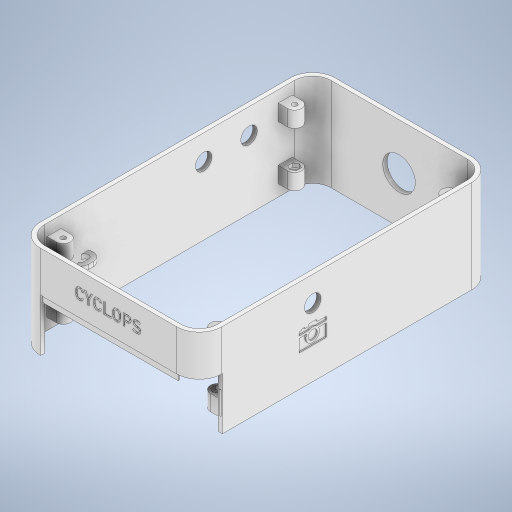
# Autodesk Inventor part: MIDDLE
Saved by Autodesk Inventor 2023 (Build 270158000, 158)
## iProperties
Created: 2023-03-14
Part Number: MIDDLE
Material: PC/ABS Plastic
Document SubType Name: Modeling
Designer: Amos Yu
Density: 0.357273 g/cm^3
Appearance: White
Author: Amos Yu
Autodesk Inventor part; units mm, degrees
note: some values were not read from the file. Chosen so that the rebuilt part matches the saved one: direction of "Hole2"; direction of "Hole3"; direction of "Hole4".
ref_plane "YZ Plane" through (0, 0, 0) normal (1, 0, 0) x (0, 1, 0)
sketch "Sketch1" plane through (0, 0, 0) normal (0, 1, 0) x (-1, 0, 0)
  line L0 (10, 0) -> (70, 0)
  line L1 (80, -10) -> (80, -120)
  line L2 (70, -130) -> (10, -130)
  line L3 (0, -120) -> (0, -10)
  arc A0 (80, -10) -> (70, 0) centre (70, -10) ccw
  arc A1 (10, 0) -> (0, -10) centre (10, -10) ccw
  arc A2 (0, -120) -> (10, -130) centre (10, -120) ccw
  arc A3 (70, -130) -> (80, -120) centre (70, -120) ccw
  line L4 (78.1, -120) -> (78.1, -10)
  arc A4 (78.1, -10) -> (70, -1.9) centre (70, -10) ccw
  line L5 (70, -1.9) -> (10, -1.9)
  arc A5 (10, -1.9) -> (1.9, -10) centre (10, -10) ccw
  line L6 (1.9, -10) -> (1.9, -120)
  arc A6 (1.9, -120) -> (10, -128.1) centre (10, -120) ccw
  line L7 (10, -128.1) -> (70, -128.1)
  arc A7 (70, -128.1) -> (78.1, -120) centre (70, -120) ccw
  point P0 (0, 0)
  point P1 (80, -130)
  point P2 (80, 0)
  point P3 (0, -130)
  dimension "d0" = 80
  dimension "d1" = 130
  dimension "d2" = 10
  dimension "d3" = 1.9
  constraints: 16 end point, 16 point on circle, 8 centre point, 8 point on line, 8 tangent, 4 parallel, 3 equal radius, 2 perpendicular, 1 horizontal, 7 other
  measures "d0" distance of point (80, -130) point (0, -130)
  measures "d1" distance of point (80, 0) point (80, -130)
  measures "d2" radius of A0
  measures "d3" distance between parallel lines of L1 L4
extrude "Extrusion1" add sketch "Sketch1" along normal mid plane 41
ref_plane "Work Plane1" through (0, -15.4, 0) normal (0, -1, 0) x (1, 0, 0)
sketch "Sketch2" plane through (0, -15.4, 0) normal (0, -1, 0) x (1, 0, 0)
  circle A0 centre (-6, -14) radius 1.1
  arc A1 (-6, -10.9) -> (-6, -17.1) centre (-6, -14) ccw
  line L0 (-6, -10.9) -> (-1.9, -10.9)
  line L1 (-1.9, -10.9) -> (-1.9, -17.1)
  line L2 (-1.9, -17.1) -> (-6, -17.1)
  line L3 (-1.9, -120) -> (-1.9, -10) projected
  circle A2 centre (-6, -116) radius 1.1
  arc A3 (-6, -112.9) -> (-6, -119.1) centre (-6, -116) ccw
  line L4 (-6, -112.9) -> (-1.9, -112.9)
  line L5 (-1.9, -112.9) -> (-1.9, -119.1)
  line L6 (-1.9, -119.1) -> (-6, -119.1)
  line L7 (-10, -1.9) -> (-70, -1.9) construction
  line L8 (-40, -1.9) -> (-40, -128.1) construction
  line L9 (-70, -128.1) -> (-10, -128.1) construction
  circle A4 centre (-74, -14) radius 1.1
  arc A5 (-74, -17.1) -> (-74, -10.9) centre (-74, -14) ccw
  line L10 (-74, -10.9) -> (-78.1, -10.9)
  line L11 (-78.1, -10.9) -> (-78.1, -17.1)
  line L12 (-78.1, -17.1) -> (-74, -17.1)
  circle A6 centre (-74, -116) radius 1.1
  arc A7 (-74, -119.1) -> (-74, -112.9) centre (-74, -116) ccw
  line L13 (-74, -112.9) -> (-78.1, -112.9)
  line L14 (-78.1, -112.9) -> (-78.1, -119.1)
  line L15 (-78.1, -119.1) -> (-74, -119.1)
  point P0 (0, 0)
  point P1 (-78.1, -120)
  point P2 (-78.1, -10)
  point P3 (-1.9, -119.1)
  point P4 (-1.9, -112.9)
  dimension "d7" = 2.2
  dimension "d8" = 14
  dimension "d9" = 6
  dimension "d10" = 2
  dimension "d13" = 102
  constraints: 26 end point, 14 symmetric about line, 8 centre point, 8 point on circle, 4 coincident, 2 midpoint, 2 tangent, 2 vertical, 1 collinear, 1 horizontal, 1 parallel, 15 other
  measures "d7" diameter of A0
  measures "d8" vertical distance of point (0, 0) A0.centre
  measures "d9" horizontal distance of A0.centre point (0, 0)
  measures "d10" radial gap between concentric circles of A0 A1
  measures "d13" distance of A0.centre A2.centre
extrude "Extrusion2" add sketch "Sketch2" against normal blind 7
sketch "Sketch11" plane through (0, -8.4, 0) normal (0, 1, 0) x (1, 0, 0)
  circle A0 centre (-6, 14) radius 1.1 construction
  line L0 (-7.9, 15.097) -> (-6, 16.1939)
  line L1 (-6, 16.1939) -> (-4.1, 15.097)
  line L2 (-4.1, 15.097) -> (-4.1, 12.903)
  line L3 (-4.1, 12.903) -> (-6, 11.8061)
  line L4 (-6, 11.8061) -> (-7.9, 12.903)
  line L5 (-7.9, 12.903) -> (-7.9, 15.097)
  line L6 (-70, 0) -> (-10, 0) construction
  line L7 (0, 10) -> (0, 120) construction
  line L8 (-75.9, 15.097) -> (-74, 16.1939)
  line L9 (-74, 16.1939) -> (-72.1, 15.097)
  line L10 (-72.1, 15.097) -> (-72.1, 12.903)
  line L11 (-72.1, 12.903) -> (-74, 11.8061)
  line L12 (-74, 11.8061) -> (-75.9, 12.903)
  line L13 (-75.9, 12.903) -> (-75.9, 15.097)
  line L14 (-7.9, 117.097) -> (-6, 118.1939)
  line L15 (-6, 118.1939) -> (-4.1, 117.097)
  line L16 (-4.1, 117.097) -> (-4.1, 114.903)
  line L17 (-4.1, 114.903) -> (-6, 113.8061)
  line L18 (-6, 113.8061) -> (-7.9, 114.903)
  line L19 (-7.9, 114.903) -> (-7.9, 117.097)
  line L20 (-75.9, 117.097) -> (-74, 118.1939)
  line L21 (-74, 118.1939) -> (-72.1, 117.097)
  line L22 (-72.1, 117.097) -> (-72.1, 114.903)
  line L23 (-72.1, 114.903) -> (-74, 113.8061)
  line L24 (-74, 113.8061) -> (-75.9, 114.903)
  line L25 (-75.9, 114.903) -> (-75.9, 117.097)
  point P0 (0, 0)
  dimension "d68" = 1.9
  dimension "d71" = 68
  dimension "d74" = 102
  constraints: 48 end point, 2 vertical, 1 coincident, 1 horizontal, 49 other
  measures "d68" distance from line of L5 point (-6, 14)
  measures "d71" distance of L0.start L8.start
  measures "d74" distance of L0.start L14.start
extrude "Extrusion6" cut sketch "Sketch11" against normal blind 1.7
mirror "Mirror1" about plane through (0, 0, 0) normal (0, 1, 0) of "Extrusion2", "Extrusion6"
sketch "Sketch4" plane through (-80, -20.5, -10) normal (-1, 0, 0) x (0, 0, 1)
  line L0 (0, 0) -> (-110, 0) projected
  point P0 (10, 20.5)
  point P1 (-70, 30)
  point P2 (-90, 30)
  dimension "d34" = 80
  dimension "d35" = 100
  dimension "d36" = 30
  constraints: 1 horizontal alignment
  measures "d34" horizontal distance of point (10, 20.5) point (-70, 30)
  measures "d35" horizontal distance of point (-90, 30) point (10, 20.5)
  measures "d36" distance from line of L0 point (-70, 30)
hole "Hole2" at (-80, 9.5, -80) at (-80, 9.5, -100) direction (1, 0, 0) diameter 7.2 depth 1.9
sketch "Sketch5" plane through (0, -20.5, -120) normal (1, 0, 0) x (0, 0, -1)
  line L0 (0, 0) -> (-110, 0) projected
  point P0 (-120, 20.5)
  point P1 (-70, 30)
  dimension "d44" = 50
  dimension "d45" = 30
  measures "d44" horizontal distance of point (-120, 20.5) point (-70, 30)
  measures "d45" distance from line of L0 point (-70, 30)
hole "Hole3" at (0, 9.5, -50) direction (-1, 0, 0) diameter 7.2 depth 1.9
sketch "Sketch6" plane through (-10, 20.5, -130) normal (0, 0, -1) x (-1, 0, 0)
  line L0 (60, -41) -> (0, -41) projected
  line L1 (0, 0) -> (60, 0) projected
  line L2 (60, 0) -> (0, 0) construction
  line L3 (30, 0) -> (30, -41) construction
  point P0 (-10, -20.5)
  point P1 (30, -20.5)
  point P2 (30, -20.5)
  constraints: 3 midpoint, 2 end point, 1 coincident
hole "Hole4" at (-40, 0, -130) direction (0, 0, 1) diameter 14.3 depth 1.9
sketch "Sketch7" plane through (0, 0, 0) normal (0, 0, 1) x (1, 0, 0)
  line L0 (-70, 2.5) -> (0, 2.5)
  line L1 (0, 2.5) -> (0, -20.5)
  line L2 (0, -20.5) -> (-70, -20.5)
  line L3 (-70, -20.5) -> (-70, 2.5)
  line L4 (0, -20.5) -> (0, 20.5) projected
  line L5 (-10, -20.5) -> (-70, -20.5) projected
  point P0 (0, 0)
  dimension "d53" = 70
  dimension "d57" = 23
  constraints: 8 end point, 2 collinear, 2 parallel, 1 horizontal, 1 perpendicular
  measures "d53" distance of L1.end L2.end
  measures "d57" distance of L0.end L1.end
extrude "Extrusion3" cut sketch "Sketch7" against normal blind 10.2
sketch "Sketch8" plane through (-70, -20.5, -1.9) normal (1, 0, 0) x (0, 0, -1)
  line L0 (-1.2, 23) -> (-0.7, 23)
  line L1 (-0.7, 23) -> (-0.7, 20)
  line L2 (-0.7, 20) -> (-1.2, 20)
  line L3 (-1.2, 20) -> (-1.2, 23)
  line L4 (-1.9, 23) -> (0, 23) projected
  point P0 (-1.9, 20.5)
  point P1 (-0.95, 23)
  dimension "d58" = 0.5
  dimension "d59" = 3
  constraints: 8 end point, 2 midpoint, 2 parallel, 1 horizontal, 1 perpendicular
  measures "d58" distance of L1.end L2.end
  measures "d59" distance of L0.end L1.end
extrude "Extrusion4" add sketch "Sketch8" along normal blind 60
ref_plane "Work Plane2" through (0, -9, 0) normal (0, -1, 0) x (1, 0, 0)
sketch "Sketch10" plane through (0, -9, 0) normal (0, -1, 0) x (1, 0, 0)
  line L0 (0, -10.2) -> (-1.9, -10.2) projected
  arc A0 (-0.517, -10.2) -> (-1.383, -10.2) centre (-0.95, -10.45) ccw
  point P0 (0, 0)
  point P1 (-0.95, -9.95)
  point P2 (-0.95, -10.2)
  dimension "d63" = 0.5
  dimension "d65" = 0.25
  constraints: 3 point on circle, 2 point on line, 1 centre point, 1 midpoint, 1 vertical alignment
  measures "d63" radius of A0
  measures "d65" distance from line of A0.centre L0
extrude "Extrusion5" add sketch "Sketch10" along normal mid plane 10
sketch "Sketch12" plane through (0, 0, 0) normal (0, 1, 0) x (-1, 0, 0)
  line L0 (76.45, -24) -> (76.45, -26) construction
  line L1 (74.8, -24) -> (74.8, -26)
  arc A0 (74.8, -26) -> (78.1, -26) centre (76.45, -26) ccw
  line L2 (76.45, -24) -> (76.45, -26) construction
  line L3 (72.8, -24) -> (72.8, -26)
  arc A1 (74.9074, -20.692) -> (72.8, -24) centre (76.45, -24) ccw
  arc A2 (72.8, -26) -> (78.1, -29.2558) centre (76.45, -26) ccw
  line L4 (78.1, -26) -> (78.1, -29.2558)
  line L5 (75.7527, -22.5046) -> (74.9074, -20.692)
  line L6 (78.1, -120) -> (78.1, -10) projected
  arc A3 (75.7527, -22.5046) -> (74.8, -24) centre (76.45, -24) ccw
  point P0 (0, 0)
  point P1 (76.45, -25)
  point P2 (76.45, -25)
  point P3 (76.45, -22.35)
  point P4 (76.45, -27.65)
  dimension "d85" = 2
  dimension "d88" = 3.3
  dimension "d89" = 25
  dimension "d90" = 25
  dimension "d91" = 5.3
  constraints: 16 end point, 10 point on circle, 5 tangent, 4 centre point, 2 collinear, 2 midpoint, 2 vertical, 1 parallel, 1 point on line, 1 vertical alignment
  measures "d85" distance between parallel lines of L3 L1
  measures "d88" diameter of A0
  measures "d89" vertical distance of point (0, 0) point (76.45, -25)
  measures "d90" angle of L6 L5
  measures "d91" distance of point (76.45, -27.65) point (76.45, -22.35)
extrude "Extrusion7" add sketch "Sketch12" along normal mid plane 2
sketch "Sketch15" plane through (-70, 20.5, 0) normal (0, 0, 1) x (1, 0, 0)
  line L0 (15, -6.25) -> (45, -6.25) construction
  line L1 (45, -6.25) -> (45, -11.75) construction
  line L2 (45, -11.75) -> (15, -11.75) construction
  line L3 (15, -11.75) -> (15, -6.25) construction
  line L4 (0, 0) -> (60, 0) projected
  line L5 (0, -18) -> (0, 0) projected
  spline S0 degree 2 poles (17.2543, -11.3532) (16.7382, -11.3532) (15.9496, -10.8949) (15.5161, -10.0485) (15.5161, -9.4911) knots 0 0 0 1 2 3 3 3
  line L6 (15.5161, -9.4911) -> (15.5161, -8.1204)
  spline S1 degree 2 poles (15.5161, -8.1204) (15.5161, -7.563) (15.9496, -6.7166) (16.7382, -6.25) (17.2543, -6.25) knots 0 0 0 1 2 3 3 3
  spline S2 degree 2 poles (17.2543, -6.25) (17.6879, -6.25) (18.4104, -6.6175) (18.8935, -7.2946) (18.9802, -7.7364) knots 0 0 0 1 2 3 3 3
  line L7 (18.9802, -7.7364) -> (18.2618, -7.7364)
  spline S3 degree 2 poles (18.2618, -7.7364) (18.1957, -7.5052) (17.8902, -7.1336) (17.4773, -6.9354) (17.2543, -6.9354) knots 0 0 0 1 2 3 3 3
  spline S4 degree 2 poles (17.2543, -6.9354) (16.9488, -6.9354) (16.4905, -7.2327) (16.2345, -7.7653) (16.2345, -8.1204) knots 0 0 0 1 2 3 3 3
  line L8 (16.2345, -8.1204) -> (16.2345, -9.4911)
  spline S5 degree 2 poles (16.2345, -9.4911) (16.2345, -9.8421) (16.4905, -10.3788) (16.9488, -10.672) (17.2543, -10.672) knots 0 0 0 1 2 3 3 3
  spline S6 degree 2 poles (17.2543, -10.672) (17.4814, -10.672) (17.8902, -10.4862) (18.1957, -10.1187) (18.2618, -9.871) knots 0 0 0 1 2 3 3 3
  line L9 (18.2618, -9.871) -> (18.9802, -9.871)
  spline S7 degree 2 poles (18.9802, -9.871) (18.8935, -10.3128) (18.4063, -10.9858) (17.6837, -11.3532) (17.2543, -11.3532) knots 0 0 0 1 2 3 3 3
  line L10 (21.4822, -9.2723) -> (21.4822, -11.3037)
  line L11 (21.4822, -11.3037) -> (20.7803, -11.3037)
  line L12 (20.7803, -11.3037) -> (20.7803, -9.2723)
  line L13 (20.7803, -9.2723) -> (19.2568, -6.3037)
  line L14 (19.2568, -6.3037) -> (20.0372, -6.3037)
  line L15 (20.0372, -6.3037) -> (21.1313, -8.558)
  line L16 (21.1313, -8.558) -> (22.2254, -6.3037)
  line L17 (22.2254, -6.3037) -> (23.0058, -6.3037)
  line L18 (23.0058, -6.3037) -> (21.4822, -9.2723)
  spline S8 degree 2 poles (25.1569, -11.3532) (24.6408, -11.3532) (23.8522, -10.8949) (23.4187, -10.0485) (23.4187, -9.4911) knots 0 0 0 1 2 3 3 3
  line L19 (23.4187, -9.4911) -> (23.4187, -8.1204)
  spline S9 degree 2 poles (23.4187, -8.1204) (23.4187, -7.563) (23.8522, -6.7166) (24.6408, -6.25) (25.1569, -6.25) knots 0 0 0 1 2 3 3 3
  spline S10 degree 2 poles (25.1569, -6.25) (25.5904, -6.25) (26.313, -6.6175) (26.796, -7.2946) (26.8827, -7.7364) knots 0 0 0 1 2 3 3 3
  line L20 (26.8827, -7.7364) -> (26.1643, -7.7364)
  spline S11 degree 2 poles (26.1643, -7.7364) (26.0983, -7.5052) (25.7927, -7.1336) (25.3799, -6.9354) (25.1569, -6.9354) knots 0 0 0 1 2 3 3 3
  spline S12 degree 2 poles (25.1569, -6.9354) (24.8514, -6.9354) (24.3931, -7.2327) (24.1371, -7.7653) (24.1371, -8.1204) knots 0 0 0 1 2 3 3 3
  line L21 (24.1371, -8.1204) -> (24.1371, -9.4911)
  spline S13 degree 2 poles (24.1371, -9.4911) (24.1371, -9.8421) (24.3931, -10.3788) (24.8514, -10.672) (25.1569, -10.672) knots 0 0 0 1 2 3 3 3
  spline S14 degree 2 poles (25.1569, -10.672) (25.384, -10.672) (25.7927, -10.4862) (26.0983, -10.1187) (26.1643, -9.871) knots 0 0 0 1 2 3 3 3
  line L22 (26.1643, -9.871) -> (26.8827, -9.871)
  spline S15 degree 2 poles (26.8827, -9.871) (26.796, -10.3128) (26.3088, -10.9858) (25.5863, -11.3532) (25.1569, -11.3532) knots 0 0 0 1 2 3 3 3
  line L23 (27.8819, -6.3037) -> (28.5838, -6.3037)
  line L24 (28.5838, -6.3037) -> (28.5838, -11.3037)
  line L25 (28.5838, -11.3037) -> (27.8819, -11.3037)
  line L26 (27.8819, -11.3037) -> (27.8819, -6.3037)
  line L27 (28.2329, -10.6348) -> (31.0941, -10.6348)
  line L28 (31.0941, -10.6348) -> (31.0941, -11.3037)
  line L29 (31.0941, -11.3037) -> (28.2329, -11.3037)
  line L30 (28.2329, -11.3037) -> (28.2329, -10.6348)
  spline S16 degree 2 poles (33.5756, -11.3532) (33.0512, -11.3532) (32.2543, -10.8991) (31.8167, -10.0609) (31.8167, -9.5118) knots 0 0 0 1 2 3 3 3
  line L31 (31.8167, -9.5118) -> (31.8167, -8.0956)
  spline S17 degree 2 poles (31.8167, -8.0956) (31.8167, -7.5464) (32.2543, -6.7083) (33.0512, -6.25) (33.5756, -6.25) knots 0 0 0 1 2 3 3 3
  spline S18 degree 2 poles (33.5756, -6.25) (34.0958, -6.25) (34.8968, -6.7083) (35.3303, -7.5464) (35.3303, -8.0956) knots 0 0 0 1 2 3 3 3
  line L32 (35.3303, -8.0956) -> (35.3303, -9.5118)
  spline S19 degree 2 poles (35.3303, -9.5118) (35.3303, -10.0609) (34.8968, -10.8991) (34.0958, -11.3532) (33.5756, -11.3532) knots 0 0 0 1 2 3 3 3
  spline S20 degree 2 poles (33.5756, -10.6637) (33.8852, -10.6637) (34.3559, -10.3871) (34.6119, -9.871) (34.6119, -9.5365) knots 0 0 0 1 2 3 3 3
  line L33 (34.6119, -9.5365) -> (34.6119, -8.0708)
  spline S21 degree 2 poles (34.6119, -8.0708) (34.6119, -7.7322) (34.3559, -7.2203) (33.8852, -6.9436) (33.5756, -6.9436) knots 0 0 0 1 2 3 3 3
  spline S22 degree 2 poles (33.5756, -6.9436) (33.2659, -6.9436) (32.7952, -7.2203) (32.5351, -7.7322) (32.5351, -8.0708) knots 0 0 0 1 2 3 3 3
  line L34 (32.5351, -8.0708) -> (32.5351, -9.5365)
  spline S23 degree 2 poles (32.5351, -9.5365) (32.5351, -9.871) (32.7952, -10.3871) (33.2659, -10.6637) (33.5756, -10.6637) knots 0 0 0 1 2 3 3 3
  line L35 (36.8249, -8.6984) -> (38.4269, -8.6984)
  spline S24 degree 2 poles (38.4269, -8.6984) (38.654, -8.6984) (38.9967, -8.4837) (39.1866, -8.0915) (39.1866, -7.8355) knots 0 0 0 1 2 3 3 3
  spline S25 degree 2 poles (39.1866, -7.8355) (39.1866, -7.5795) (38.9967, -7.1872) (38.654, -6.9684) (38.4269, -6.9684) knots 0 0 0 1 2 3 3 3
  line L36 (38.4269, -6.9684) -> (36.8249, -6.9684)
  line L37 (36.8249, -6.9684) -> (36.8249, -6.3037)
  line L38 (36.8249, -6.3037) -> (38.4021, -6.3037)
  spline S26 degree 2 poles (38.4021, -6.3037) (38.8481, -6.3037) (39.5293, -6.6835) (39.905, -7.3813) (39.905, -7.8355) knots 0 0 0 1 2 3 3 3
  spline S27 degree 2 poles (39.905, -7.8355) (39.905, -8.2938) (39.5293, -8.9874) (38.8481, -9.3631) (38.4021, -9.3631) knots 0 0 0 1 2 3 3 3
  line L39 (38.4021, -9.3631) -> (36.8249, -9.3631)
  line L40 (36.8249, -9.3631) -> (36.8249, -8.6984)
  line L41 (36.4657, -6.3037) -> (37.1676, -6.3037)
  line L42 (37.1676, -6.3037) -> (37.1676, -11.3037)
  line L43 (37.1676, -11.3037) -> (36.4657, -11.3037)
  line L44 (36.4657, -11.3037) -> (36.4657, -6.3037)
  spline S28 degree 2 poles (42.3534, -11.3532) (41.9942, -11.3532) (41.346, -11.217) (40.7845, -10.9445) (40.5409, -10.738) knots 0 0 0 1 2 3 3 3
  line L45 (40.5409, -10.738) -> (40.9785, -10.2013)
  spline S29 degree 2 poles (40.9785, -10.2013) (41.2634, -10.449) (41.9529, -10.6967) (42.3534, -10.6967) knots 0 0 0 1 2 2 2
  spline S30 degree 2 poles (42.3534, -10.6967) (42.8984, -10.6967) (43.4971, -10.2921) (43.4971, -9.9246) knots 0 0 0 1 2 2 2
  line L46 (43.4971, -9.9246) -> (43.4971, -9.9205)
  spline S31 degree 2 poles (43.4971, -9.9205) (43.4971, -9.6604) (43.2246, -9.3549) (42.7952, -9.2062) (42.4525, -9.1443) knots 0 0 0 1 2 3 3 3
  spline S32 degree 2 poles (42.4525, -9.1443) (42.4443, -9.1402) (42.4195, -9.1402) (42.4071, -9.136) knots 0 0 0 1 2 2 2
  line L47 (42.4071, -9.136) -> (42.3576, -9.1278)
  spline S33 degree 2 poles (42.3576, -9.1278) (41.8538, -9.0411) (41.2263, -8.8223) (40.7762, -8.2483) (40.7762, -7.7199) knots 0 0 0 1 2 3 3 3
  line L48 (40.7762, -7.7199) -> (40.7762, -7.7157)
  spline S34 degree 2 poles (40.7762, -7.7157) (40.7762, -7.2533) (41.1932, -6.5968) (41.9942, -6.25) (42.5516, -6.25) knots 0 0 0 1 2 3 3 3
  spline S35 degree 2 poles (42.5516, -6.25) (42.82, -6.25) (43.3402, -6.3697) (43.8439, -6.5968) (44.0917, -6.7744) knots 0 0 0 1 2 3 3 3
  line L49 (44.0917, -6.7744) -> (43.6912, -7.3318)
  spline S36 degree 2 poles (43.6912, -7.3318) (43.4063, -7.1212) (42.8365, -6.9106) (42.5516, -6.9106) knots 0 0 0 1 2 2 2
  spline S37 degree 2 poles (42.5516, -6.9106) (42.0396, -6.9106) (41.474, -7.3194) (41.474, -7.6951) knots 0 0 0 1 2 2 2
  line L50 (41.474, -7.6951) -> (41.474, -7.6992)
  spline S38 degree 2 poles (41.474, -7.6992) (41.474, -7.9552) (41.7671, -8.2525) (42.2007, -8.3929) (42.5888, -8.4713) knots 0 0 0 1 2 3 3 3
  spline S39 degree 2 poles (42.5888, -8.4713) (42.6053, -8.4713) (42.6301, -8.4754) (42.6424, -8.4796) knots 0 0 0 1 2 2 2
  spline S40 degree 2 poles (42.6424, -8.4796) (42.659, -8.4837) (42.7002, -8.4919) (42.7168, -8.4919) knots 0 0 0 1 2 2 2
  spline S41 degree 2 poles (42.7168, -8.4919) (43.1709, -8.5869) (43.782, -8.8429) (44.1908, -9.4085) (44.1908, -9.8999) knots 0 0 0 1 2 3 3 3
  line L51 (44.1908, -9.8999) -> (44.1908, -9.9081)
  spline S42 degree 2 poles (44.1908, -9.9081) (44.1908, -10.3664) (43.7572, -11.0147) (42.9356, -11.3532) (42.3534, -11.3532) knots 0 0 0 1 2 3 3 3
  point P0 (70, -20.5)
  point P1 (30, -6.25)
  point P2 (30, 0)
  point P3 (15, -9)
  point P4 (0, -9)
  dimension "d127" = 30
  dimension "d128" = 5.5
  constraints: 4 midpoint, 1 horizontal, 1 horizontal alignment, 1 vertical alignment, 2 other
  measures "d127" distance of L0.start L0.end
  measures "d128" distance of L0.end L1.end
emboss "Emboss3" sketch "Sketch15" operation cut depth 0.5 direction (0, 0, -1) contours S0 L6 S1 S2 L7 S3 S4 L8 S5 S6 L9 S7 | L10 L11 L12 L13 L14 L15 L16 L17 L18 | S8 L19 S9 S10 L20 S11 S12 L21 S13 S14 L22 S15 | L23 L24 L27 L30 L25 L26 | L27 L28 L29 L24 | L24 L25 L30 L27 | S16 L31 S17 S18 L32 S19 | L40 L39 L42 L43 L44 L41 L37 L36 L35 | L35 L42 L39 L40 | L35 S24 S25 L36 L42 L38 S26 S27 L39 | L36 L37 L38 L42 | S28 L45 S29 S30 L46 S31 S32 L47 S33 L48 S34 S35 L49 S36 S37 L50 S38 S39 S40 S41 L51 S42
sketch "Sketch13" plane through (0, -20.5, -120) normal (1, 0, 0) x (0, 0, -1)
  circle A0 centre (-70, 30) radius 3.6 projected
  line L0 (-76, 14) -> (-64, 14)
  line L1 (-72.0774, 22) -> (-71.5, 23)
  line L2 (-71.5, 23) -> (-68.5, 23)
  line L3 (-68.5, 23) -> (-67.9226, 22)
  circle A1 centre (-70, 18) radius 2
  line L4 (-64, 22) -> (-67.9226, 22)
  line L5 (-76, 19.5) -> (-72.5981, 19.5)
  line L6 (-67.4019, 19.5) -> (-64, 19.5)
  line L7 (-76, 20.5) -> (-71.6583, 20.5)
  line L8 (-68.3417, 20.5) -> (-64, 20.5)
  arc A2 (-72.5981, 19.5) -> (-67.4019, 19.5) centre (-70, 18) ccw
  arc A3 (-68.3417, 20.5) -> (-71.6583, 20.5) centre (-70, 18) ccw
  line L9 (-64, 14) -> (-64, 19.5)
  line L10 (-64, 20.5) -> (-64, 22)
  line L11 (-76, 22) -> (-76, 20.5)
  line L12 (-76, 19.5) -> (-76, 14)
  line L13 (-75, 22) -> (-75, 22.5)
  line L14 (-75, 22.5) -> (-73.5, 22.5)
  line L15 (-73.5, 22.5) -> (-73.5, 22)
  line L16 (-72.0774, 22) -> (-73.5, 22)
  line L17 (-75, 22) -> (-76, 22)
  point P0 (-120, 20.5)
  point P1 (-70, 23)
  point P2 (-70, 14)
  point P3 (-64, 18)
  dimension "d92" = 12
  dimension "d93" = 4
  dimension "d95" = 12
  dimension "d96" = 8
  dimension "d97" = 3
  dimension "d99" = 1
  dimension "d102" = 1.5
  dimension "d103" = 1
  dimension "d104" = 3
  dimension "d105" = 3
  dimension "d106" = 120
  dimension "d108" = 4
  dimension "d110" = 1.5
  dimension "d111" = 0.5
  dimension "d112" = 1
  dimension "d113" = 120
  constraints: 36 end point, 21 perpendicular, 5 vertical alignment, 4 horizontal alignment, 4 parallel, 4 point on circle, 3 centre point, 3 vertical, 2 midpoint, 1 coincident, 1 point on line
  measures "d92" distance of A0.centre A2.centre
  measures "d93" diameter of A1
  measures "d95" distance of L0.start L0.end
  measures "d96" distance of L0.end L4.start
  measures "d97" distance of L1.end L2.end
  measures "d99" distance between parallel lines of L4 L2
  measures "d102" distance between parallel lines of L4 L8
  measures "d103" distance between parallel lines of L8 L6
  measures "d104" radius of A2
  measures "d105" radius of A3
  measures "d106" angle of L4 L3
  measures "d108" distance from line of A2.centre L0
  measures "d110" distance of L13.end L14.end
  measures "d111" distance of L13.start L13.end
  measures "d112" distance of L13.start L11.start
  measures "d113" angle of L16 L1
emboss "Emboss1" sketch "Sketch13" operation cut depth 0.5 direction (-1, 0, 0) contours L12 L5 A2 L6 L9 L0 | L1 L2 L3 L4 L10 L8 A3 L7 L11 L17 L13 L14 L15 L16 | A1
sketch "Sketch14" plane through (-80, -20.5, -10) normal (-1, 0, 0) x (0, 0, 1)
  circle A0 centre (-90, 30) radius 3.6 projected
  circle A1 centre (-70, 30) radius 3.6 projected
  line L0 (-90.65, 22.5) -> (-89.35, 22.5)
  line L1 (-89.35, 22.5) -> (-89.35, 13.5)
  line L2 (-89.35, 13.5) -> (-90.65, 13.5)
  line L3 (-90.65, 13.5) -> (-90.65, 22.5)
  line L4 (-90.65, 22.5) -> (-89.35, 13.5) construction
  line L5 (-89.35, 22.5) -> (-90.65, 13.5) construction
  line L6 (-70, 16.5) -> (-70, 19.5) construction
  line L7 (-67, 16.5) -> (-67, 19.5)
  line L8 (-73, 19.5) -> (-73, 16.5)
  arc A2 (-73, 16.5) -> (-67, 16.5) centre (-70, 16.5) ccw
  arc A3 (-67, 19.5) -> (-73, 19.5) centre (-70, 19.5) ccw
  line L9 (-70, 19.5) -> (-70, 16.5) construction
  line L10 (-71.7, 19.5) -> (-71.7, 16.5)
  line L11 (-68.3, 16.5) -> (-68.3, 19.5)
  arc A4 (-68.3, 19.5) -> (-71.7, 19.5) centre (-70, 19.5) ccw
  arc A5 (-71.7, 16.5) -> (-68.3, 16.5) centre (-70, 16.5) ccw
  point P0 (10, 20.5)
  point P1 (-90, 18)
  point P2 (-70, 18)
  point P3 (-70, 18)
  point P4 (-70, 22.5)
  point P5 (-70, 13.5)
  dimension "d116" = 12
  dimension "d117" = 9
  dimension "d118" = 1.3
  dimension "d119" = 12
  dimension "d120" = 9
  dimension "d121" = 1.3
  dimension "d122" = 6
  constraints: 28 end point, 10 point on circle, 8 tangent, 5 equal length, 4 centre point, 4 midpoint, 2 vertical alignment, 1 horizontal, 1 perpendicular, 1 vertical
  measures "d116" distance of A0.centre point (-90, 18)
  measures "d117" distance of L0.end L1.end
  measures "d118" distance of L0.start L0.end
  measures "d119" distance of A1.centre point (-70, 18)
  measures "d120" distance of point (-70, 22.5) point (-70, 13.5)
  measures "d121" distance between parallel lines of L7 L11
  measures "d122" distance of L7.end L8.start
emboss "Emboss2" sketch "Sketch14" operation cut depth 0.5 direction (1, 0, 0) contours L0 L1 L2 L3 | A2 L8 A3 L7
sketch "Sketch34" plane through (0, -20.5, 0) normal (0, -1, 0) x (1, 0, 0)
  line L0 (22.6612, -156.3383) -> (-108.8757, -156.3383)
  line L1 (-108.8757, -156.3383) -> (-108.8757, 14.6597)
  line L2 (-108.8757, 14.6597) -> (22.6612, 14.6597)
  line L3 (22.6612, 14.6597) -> (22.6612, -156.3383)
  point P0 (0, 0)
  constraints: 8 end point, 2 parallel, 1 horizontal, 1 perpendicular
equation "\"d2\" = fillet_outer_radius"
equation "\"d3\" = thickness - tol"
equation "\"d4\" = total_height - 2 * thickness"
equation "\"d7\" = bolt_thread_diameter + 2 * tol"
equation "\"d8\" = bolt_inset_depth"
equation "\"d9\" = bolt_inset_width"
equation "\"d10\" = thickness"
equation "\"d13\" = total_depth - 2 * bolt_inset_depth"
equation "\"d18\" = bolt_housing_height"
equation "\"d68\" = 0.5 * nut_width - tol"
equation "\"d71\" = total_width - 2 * bolt_inset_width"
equation "\"d74\" = total_depth - 2 * bolt_inset_depth"
equation "\"d77\" = nut_height + tol"
equation "\"d34\" = button_off_depth"
equation "\"d35\" = button_on_depth"
equation "\"d36\" = button_height"
equation "\"d27\" = button_thread_diameter + 2 * tol"
equation "\"d44\" = button_capture_depth"
equation "\"d45\" = button_height"
equation "\"d37\" = button_thread_diameter + 2 * tol"
equation "\"d46\" = camera_lens_diameter + 2 * tol"
equation "\"d53\" = total_width - fillet_outer_radius"
equation "\"d57\" = door_height"
equation "\"d55\" = fillet_outer_radius + 2 * tol"
equation "\"d58\" = door_rail_depth"
equation "\"d59\" = door_rail_height"
equation "\"d60\" = total_width - 2 * fillet_outer_radius"
equation "\"d63\" = door_strike_radius"
equation "\"d66\" = door_strike_height"
equation "\"d85\" = thickness"
equation "\"d88\" = usbc_cable_diameter - 2 * tol"
equation "\"d89\" = usbc_hole_inset_depth"
equation "\"d91\" = lidar_cable_diameter + usbc_cable_diameter - 2 * tol"
equation "\"d83\" = thickness"
equation "\"d0\" = total_width"
equation "\"d1\" = total_depth"
equation "\"d125\" = emboss_thickness"
equation "\"d92\" = emboss_offset_height"
equation "\"d114\" = emboss_thickness"
equation "\"d116\" = emboss_offset_height"
equation "\"d119\" = emboss_offset_height"
equation "\"d123\" = emboss_thickness"
equation "\"bolt_housing_height\" = 7"
equation "\"d6\" = -lip_height - tol"
equation "\"button_thread_diameter\" = 7"
equation "\"button_on_depth\" = 100"
equation "\"button_off_depth\" = 80"
equation "\"button_height\" = 30"
equation "\"button_capture_depth\" = 50"
equation "\"camera_lens_diameter\" = 14.1"
equation "\"d62\" = -0.5 * door_height"
equation "\"usbc_cable_diameter\" = 3.5"
equation "\"lidar_cable_diameter\" = 2"
equation "\"emboss_offset_height\" = 12"
equation "\"emboss_thickness\" = 0.5"
equation "\"fillet_outer_radius\" = 10"
equation "\"thickness\" = 2"
equation "\"tol\" = 0.1"
equation "\"total_height\" = 45"
equation "\"bolt_thread_diameter\" = 2"
equation "\"total_depth\" = 130"
equation "\"bolt_inset_depth\" = 14"
equation "\"total_width\" = 80"
equation "\"bolt_inset_width\" = 6"
equation "\"nut_height\" = 1.6"
equation "\"door_height\" = 23"
equation "\"door_rail_depth\" = 0.5"
equation "\"door_rail_height\" = 3"
equation "\"door_strike_radius\" = 0.5"
equation "\"door_strike_height\" = 10"
equation "\"lip_height\" = 5"
equation "\"nut_width\" = 4"
equation "\"usbc_hole_inset_depth\" = 25"
body "Solid1"
